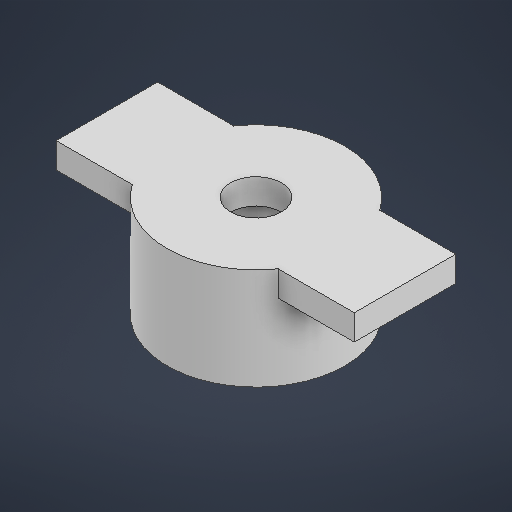
# Autodesk Inventor part: SistemLiberacion1
Saved by Autodesk Inventor 2026.1 (Build 301233000, 233)
## iProperties
Created: 2025-11-10
Part Number: SistemLiberacion1
Material: Genérico
Document SubType Name: Modeling
Designer: vickh
Density: 1 g/cm^3
Appearance: Valor por defecto
Author: vickh
Autodesk Inventor part; units mm, degrees
ref_plane "YZ Plane" through (0, 0, 0) normal (1, 0, 0) x (0, 1, 0)
ref_plane "XZ Plane" through (0, 0, 0) normal (0, 1, 0) x (-1, 0, 0)
ref_plane "XY Plane" through (0, 0, 0) normal (0, 0, 1) x (1, 0, 0)
sketch "Boceto1" plane through (0, 0, 0) normal (0, 1, 0) x (-1, 0, 0)
  circle A0 centre (0, 0) radius 10.5
  circle A1 centre (0, 0) radius 17.5
  dimension "d0" = 21
  dimension "d13" = 7
  constraints: 2 centre point, 2 coincident
  measures "d0" diameter of A0
  measures "d13" radial gap between concentric circles of A1 A0
extrude "Extrusión1" add sketch "Boceto1" along normal blind 15
sketch "Boceto2" plane through (0, 15, 0) normal (0, 1, 0) x (1, 0, 0)
  circle A0 centre (0, 0) radius 17.5 projected
  line L0 (-29.3614, -10) -> (-14.3614, -10)
  line L1 (-14.3614, 10) -> (-29.3614, 10)
  line L2 (-29.3614, 10) -> (-29.3614, -10)
  line L3 (-29.3614, -10) -> (-14.3614, 10) construction
  line L4 (-14.3614, -10) -> (-29.3614, 10) construction
  line L5 (29.3614, 10) -> (14.3614, 10)
  line L6 (14.3614, -10) -> (29.3614, -10)
  line L7 (29.3614, -10) -> (29.3614, 10)
  line L8 (29.3614, 10) -> (14.3614, -10) construction
  line L9 (14.3614, 10) -> (29.3614, -10) construction
  point P0 (-21.8614, 0)
  point P1 (21.8614, 0)
  point P2 (14.3614, -10)
  dimension "d4" = 20
  dimension "d6" = 15
  dimension "d9" = 360
  dimension "d14" = 15
  constraints: 20 end point, 4 midpoint, 2 point on circle, 1 horizontal, 1 parallel, 1 vertical, 21 other
  measures "d4" distance of L0.end L1.start
  measures "d6" distance of L0.start L0.end
  measures "d14" distance of L1.start L1.end
extrude "Extrusión2" add sketch "Boceto2" along normal blind 5
sketch "Boceto3" plane through (0, 20, 0) normal (0, 1, 0) x (1, 0, 0)
  circle A0 centre (0, 0) radius 5
  dimension "d15" = 10
  constraints: 1 centre point, 1 coincident
  measures "d15" diameter of A0
extrude "Extrusión3" cut sketch "Boceto3" against normal blind 5
equation "\"d14\" = d6"
